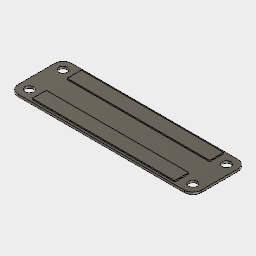
3577 PICO Hat (Autodesk Fusion 360 design; units mm, degrees)
Autodesk Fusion 360 part; units mm, degrees
sketch "Sketch1" plane through (0, 0, 0) normal (0, 0, 1) x (1, 0, 0)
  line L0 (0, 0) -> (65, 0)
  line L1 (65, 0) -> (65, 19)
  line L2 (65, 19) -> (0, 19)
  line L3 (0, 19) -> (0, 0)
  circle A0 centre (3.5, 15.5) radius 1.5
  line L4 (32.5, 19) -> (32.5, 0) construction
  line L5 (65, 9.5) -> (0, 9.5) construction
  circle A1 centre (61.5, 15.5) radius 1.5
  circle A2 centre (3.5, 3.5) radius 1.5
  circle A3 centre (61.5, 3.5) radius 1.5
  line L6 (57.77, 13.2) -> (7.23, 13.2)
  line L7 (7.23, 13.2) -> (7.23, 18.2)
  line L8 (7.23, 18.2) -> (57.77, 18.2)
  line L9 (57.77, 18.2) -> (57.77, 13.2)
  line L10 (57.77, 13.2) -> (7.23, 18.2) construction
  line L11 (7.23, 13.2) -> (57.77, 18.2) construction
  line L12 (7.23, 0.8) -> (57.77, 0.8)
  line L13 (57.77, 0.8) -> (57.77, 5.8)
  line L14 (57.77, 5.8) -> (7.23, 5.8)
  line L15 (7.23, 5.8) -> (7.23, 0.8)
  line L16 (57.77, 3.3) -> (7.23, 3.3) construction
  point P0 (32.5, 15.7)
  dimension "d1" = 65
  dimension "d2" = 19
  dimension "d3" = 3
  dimension "d4" = 3.5
  dimension "d5" = 3.5
  dimension "d6" = 50.54
  dimension "d7" = 5
  dimension "d8" = 0.8
  measures "d1" distance of L1.end L2.end
  measures "d2" distance of L0.end L1.end
  measures "d3" diameter of A0
  measures "d4" distance of L3 A0.centre
  measures "d5" distance of L2 A0.centre
  measures "d6" distance of L7.end L8.end
  measures "d7" distance of L6.end L7.end
  measures "d8" distance of L2 L8
extrude "Extrude1" add sketch "Sketch1" along normal blind 0.8 contours L0 L1 L2 L3 | L6 L7 L8 L9 | L12 L13 L14 L15
fillet "Fillet1" radius 3 4 edges at (65, 19, 0.4) (0, 0, 0.4) (65, 0, 0.4) (0, 19, 0.4)
extrude "Extrude2" add sketch "Sketch1" along normal blind 0.4 from surface at 0.8 contours L6 L7 L8 L9 | L12 L13 L14 L15
extrude "Extrude3" add sketch "Sketch1" against normal blind 0.4 contours L6 L7 L8 L9 | L12 L13 L14 L15
